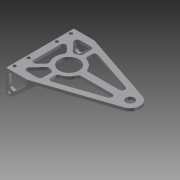
# Autodesk Inventor part: lower bix side plate 3.5
Saved by Autodesk Inventor 2012 (Build 160160000, 160)
## iProperties
Created: 2012-12-28
Part Number: lower bix side plate 3.5
Material: Default
Document SubType Name: Modeling
Designer: Bryce
Density: 1 g/cm^3
Author: Bryce
Autodesk Inventor part; units mm, degrees
ref_plane "YZ Plane" through (0, 0, 0) normal (1, 0, 0) x (0, 1, 0)
ref_plane "XZ Plane" through (0, 0, 0) normal (0, 1, 0) x (-1, 0, 0)
ref_plane "XY Plane" through (0, 0, 0) normal (0, 0, 1) x (1, 0, 0)
sketch "Sketch1" plane through (0, 0, 0) normal (0, 0, 1) x (1, 0, 0)
  line L0 (-34.925, 101.6) -> (34.925, 101.6)
  line L1 (34.925, 101.6) -> (34.925, 68.8594)
  line L2 (-34.925, 68.8594) -> (-34.925, 101.6)
  line L3 (-34.925, 68.8594) -> (-10.5309, -3.5479)
  line L4 (34.925, 68.8594) -> (10.5309, -3.5479)
  arc A0 (-10.5309, -3.5479) -> (10.5309, -3.5479) centre (0, 0) ccw
  circle A1 centre (0, 0) radius 4.7625
  circle A2 centre (0, 68.8594) radius 11.1125
  line L5 (0, 68.8594) -> (-34.925, 68.8594) construction
  line L6 (0, 68.8594) -> (34.925, 68.8594) construction
  line L7 (0, 68.8594) -> (-34.925, 101.6) construction
  line L8 (0, 68.8594) -> (34.925, 101.6) construction
  line L9 (0, 68.8594) -> (0, 0) construction
  line L10 (0, 68.8594) -> (0, 0) construction
  arc A3 (-15.6954, 66.4781) -> (-3.9688, 53.4885) centre (0, 68.8594) ccw
  arc A4 (3.9688, 53.4885) -> (15.6954, 66.4781) centre (0, 68.8594) ccw
  arc A5 (15.6954, 71.2407) -> (13.0792, 77.8566) centre (0, 68.8594) ccw
  arc A6 (9.822, 81.3311) -> (-9.822, 81.3311) centre (0, 68.8594) ccw
  arc A7 (-13.0792, 77.8566) -> (-15.6954, 71.2407) centre (0, 68.8594) ccw
  line L11 (-3.9688, 53.4885) -> (-3.9688, 10.3796)
  line L12 (3.9688, 53.4885) -> (3.9688, 10.3796)
  arc A8 (-3.9688, 10.3796) -> (-7.7188, 7.9942) centre (0, 0) ccw
  arc A9 (7.7188, 7.9942) -> (3.9688, 10.3796) centre (0, 0) ccw
  line L13 (-27.4221, 66.4781) -> (-7.7188, 7.9942)
  line L14 (7.7188, 7.9942) -> (27.4221, 66.4781)
  line L15 (-27.4221, 66.4781) -> (-15.6954, 66.4781)
  line L16 (-30.1625, 71.2407) -> (-15.6954, 71.2407)
  line L17 (15.6954, 66.4781) -> (27.4221, 66.4781)
  line L18 (15.6954, 71.2407) -> (30.1625, 71.2407)
  line L19 (-30.1625, 93.8714) -> (-13.0792, 77.8566)
  line L20 (-22.9762, 93.6625) -> (-9.822, 81.3311)
  line L21 (22.9762, 93.6625) -> (9.822, 81.3311)
  line L22 (30.1625, 93.8714) -> (13.0792, 77.8566)
  line L23 (-30.1625, 93.8714) -> (-30.1625, 71.2407)
  line L24 (-22.9762, 93.6625) -> (22.9762, 93.6625)
  line L25 (30.1625, 93.8714) -> (30.1625, 71.2407)
  arc A10 (-10.1526, 15.2183) -> (-3.9688, 16.232) centre (-7.1437, 16.232) ccw
  arc A11 (3.9688, 16.232) -> (10.1526, 15.2183) centre (7.1437, 16.232) ccw
  point P0 (-31.75, 98.425)
  point P1 (31.75, 98.425)
  point P2 (-15.875, 98.425)
  point P3 (15.875, 98.425)
  dimension "d0" = 69.85
  dimension "d1" = 101.6
  dimension "d2" = 34.925
  dimension "d6" = 18.619
  dimension "d7" = 9.525
  dimension "d8" = 32.7406
  dimension "d9" = 22.225
  dimension "d12" = 15.875
  dimension "d14" = 3.9688
  dimension "d15" = 6.35
  dimension "d16" = 6.35
  dimension "d17" = 2.3813
  dimension "d19" = 2.3813
  dimension "d22" = 2.3813
  dimension "d24" = 2.3813
  dimension "d26" = 4.7625
  dimension "d27" = 7.9375
  dimension "d28" = 4.7625
  dimension "d32" = 3.175
  dimension "d33" = 3.175
  dimension "d35" = 3.175
  dimension "d36" = 3.175
  dimension "d62" = 19.05
  dimension "d63" = 19.05
  dimension "d69" = 3.175
  dimension "d70" = 18.619
  dimension "d71" = 11.1125
  dimension "d91" = 4.7625
  dimension "d92" = 4.7625
  dimension "d93" = 4.7625
  dimension "d94" = 4.7625
  dimension "d95" = 7.9375
  constraints: 52 end point, 20 point on circle, 13 parallel, 12 centre point, 9 coincident, 7 equal radius, 7 perpendicular, 5 tangent, 4 horizontal alignment, 4 point on line, 1 collinear, 1 horizontal, 1 vertical alignment
  measures "d0" distance between parallel lines of L1 L2
  measures "d1" distance from line of point (0, 0) L0
  measures "d2" distance from line of point (0, 0) L2
  measures "d6" angle of L1 L4
  measures "d7" diameter of A1
  measures "d8" distance from line of L5.start L0
  measures "d9" diameter of A2
  measures "d12" radius of A3
  measures "d14" distance between parallel lines of L9 L12
  measures "d15" distance between parallel lines of L3 L13
  measures "d16" distance between parallel lines of L4 L14
  measures "d17" distance between parallel lines of L15 L5
  measures "d19" distance between parallel lines of L17 L6
  measures "d22" distance between parallel lines of L8 L22
  measures "d24" distance between parallel lines of L7 L19
  measures "d26" distance between parallel lines of L23 L2
  measures "d27" distance between parallel lines of L0 L24
  measures "d28" distance between parallel lines of L1 L25
  measures "d32" distance from line of L2 point (-31.75, 98.425)
  measures "d33" distance from line of L0 point (-31.75, 98.425)
  measures "d35" distance from line of L0 point (31.75, 98.425)
  measures "d36" distance from line of L1 point (31.75, 98.425)
  measures "d62" distance from line of L2 point (-15.875, 98.425)
  measures "d63" distance from line of point (15.875, 98.425) L1
  measures "d69" radius of A10
  measures "d70" angle of L3 L2
  measures "d71" radius of A0
  measures "d91" distance between parallel lines of L15 L16
  measures "d92" distance between parallel lines of L20 L19
  measures "d93" distance between parallel lines of L22 L21
  measures "d94" distance between parallel lines of L17 L18
  measures "d95" distance between parallel lines of L12 L11
extrude "Extrusion1" add sketch "Sketch1" against normal blind 3.175 contours L0 L1 L4 A0 L3 L2 | A3 L11 A10 L13 L15 | L11 A8 L13 A10 | A4 L17 L14 A11 L12 | A11 L14 A9 L12 | A5 L22 L25 L18 | A6 L20 L24 L21 | A7 L16 L23 L19
extrude "Extrusion2" cut sketch "Sketch1" against normal blind 3.175 contours A3 L11 A10 L13 L15 | A4 L17 L14 A11 L12 | A5 L22 L25 L18 | A6 L20 L24 L21 | A7 L16 L23 L19
fillet "Fillet1" radius 3.175 16 edges at (-30.1625, 71.2407, -1.5875) (-30.1625, 93.8714, -1.5875) (30.1625, 93.8714, -1.5875) (30.1625, 71.2407, -1.5875) (15.6954, 71.2407, -1.5875) (13.0792, 77.8566, -1.5875) (9.822, 81.3311, -1.5875) (-9.822, 81.3311, -1.5875) (-13.0792, 77.8566, -1.5875) (-15.6954, 71.2407, -1.5875) (15.6954, 66.4781, -1.5875) (27.4221, 66.4781, -1.5875) (3.9688, 53.4885, -1.5875) (-3.9688, 53.4885, -1.5875) (-15.6954, 66.4781, -1.5875) (-27.4221, 66.4781, -1.5875)
hole "Hole1" at (-31.75, 98.425, 0) at (31.75, 98.425, 0) at (-15.875, 98.425, 0) at (15.875, 98.425, 0) direction (0, 0, -1) diameter 3.6576 end through all
sketch "Sketch2" plane through (0, 0, 0) normal (0, 0, 1) x (1, 0, 0)
  line L0 (-22.9762, 93.6625) -> (22.9762, 93.6625) projected
  circle A0 centre (0, 68.8594) radius 11.1125 projected
  line L1 (34.925, 68.8594) -> (10.5309, -3.5479) projected
  line L2 (34.925, 101.6) -> (34.925, 68.8594) projected
  circle A1 centre (15.875, 98.425) radius 1.8288 projected
  circle A2 centre (-15.875, 98.425) radius 1.8288 projected
  circle A3 centre (-15.875, 98.425) radius 1.8288
  circle A4 centre (15.875, 98.425) radius 1.8288
  line L3 (-10.1526, 15.2183) -> (-26.0109, 62.2895) projected
  line L4 (-34.925, 101.6) -> (34.925, 101.6) projected
  line L5 (-34.925, 68.8594) -> (-38.1, 78.2835)
  line L6 (-38.1, 78.2835) -> (-38.1, 101.6)
  line L7 (-34.925, 101.6) -> (-38.1, 101.6)
  line L8 (34.925, 101.6) -> (38.1, 101.6)
  line L9 (38.1, 101.6) -> (38.1, 78.2835)
  line L10 (38.1, 78.2835) -> (34.925, 68.8594)
  line L11 (-34.925, 101.6) -> (-34.925, 68.8594)
  line L12 (34.925, 101.6) -> (34.925, 68.8594)
  dimension "d53" = 22.225
  dimension "d75" = 3.175
  dimension "d76" = 3.175
  constraints: 16 end point, 4 parallel, 2 centre point, 2 coincident, 2 collinear, 2 concentric, 2 perpendicular
  measures "d53" diameter of A0
  measures "d75" distance of L2.start L8.end
  measures "d76" distance of L4.start L6.end
fillet "Fillet6" radius 3.175 2 edges at (-22.9762, 93.6625, -1.5875) (22.9762, 93.6625, -1.5875)
extrude "Extrusion7" add sketch "Sketch2" against normal blind 25.4 contours L8 L9 L10 L2 | L5 L6 L7 L11
sketch "Sketch4" plane through (-38.1, 78.2835, 0) normal (-1, 0, 0) x (0, 0, 1)
  line L0 (-25.4, 23.3165) -> (-25.4, 0) projected
  line L1 (0, 23.3165) -> (0, 0) projected
  line L2 (0, 23.3165) -> (-25.4, 23.3165) projected
  circle A0 centre (-22.225, 20.1415) radius 1.7272
  line L3 (-25.4, 16.9665) -> (-3.9692, -7.3236)
  line L4 (-3.175, -9.4241) -> (-3.175, -81.8314) projected
  line L5 (-3.175, -9.4241) -> (-25.4, -9.4241) projected
  line L6 (-25.4, 0) -> (-25.4, -9.4241) projected
  line L7 (0, -81.8314) -> (0, 0) projected
  arc A1 (-3.175, -9.4241) -> (-3.9692, -7.3236) centre (-6.35, -9.4241) ccw
  arc A2 (-20.1746, 15.8429) -> (-17.4625, 20.1415) centre (-22.225, 20.1415) ccw
  line L8 (-20.1746, 15.8429) -> (-3.175, -3.4247)
  line L9 (-3.175, -3.4247) -> (-3.175, 20.1415)
  line L10 (-3.175, 20.1415) -> (-17.4625, 20.1415)
  point P0 (0, -78.2835)
  dimension "d79" = 3.175
  dimension "d80" = 3.175
  dimension "d81" = 3.4544
  dimension "d82" = 3.175
  dimension "d83" = 6.35
  dimension "d84" = 3.175
  dimension "d85" = 4.7625
  dimension "d86" = 3.175
  dimension "d87" = 3.175
  constraints: 8 end point, 4 point on circle, 3 centre point, 2 parallel, 2 tangent, 1 coincident, 1 perpendicular, 1 point on line
  measures "d79" distance from line of L2 A0.centre
  measures "d80" distance from line of L0 A0.centre
  measures "d81" diameter of A0
  measures "d82" radius of A1
  measures "d83" distance from line of L2 L3.start
  measures "d84" distance between parallel lines of L2 L10
  measures "d85" radius of A2
  measures "d86" distance between parallel lines of L3 L8
  measures "d87" distance between parallel lines of L1 L9
extrude "Extrusion8" cut sketch "Sketch4" against normal through all
fillet "Fillet8" radius 3.175 8 edges at (-35.9356, 74.8588, -3.175) (-36.5125, 98.425, -3.175) (-36.5125, 98.425, -17.4625) (-36.5125, 94.1265, -20.1746) (36.5125, 94.1265, -20.1746) (36.5125, 98.425, -17.4625) (36.5125, 98.425, -3.175) (35.9356, 74.8588, -3.175)
body "Solid1"
